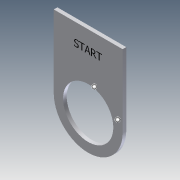
# Autodesk Inventor part: Start Button Lable
Saved by Autodesk Inventor 2016 (Build 200138000, 138)
## iProperties
Created: 2005-06-20
Part Number: Start Button Lable
Checked By: ~
Material: Generic
Document SubType Name: Modeling
Designer: BassBW
Manufacturer: Standard
Standards Organization: Custom
Density: 1 g/cm^3
Appearance: White
SCALE: 1:1
STOCK SIZE: SEE DWG
UNITS: ANSI
COMMODITY: MFG
Author: BassBW
Autodesk Inventor part; units mm, degrees
ref_plane "YZ Plane" through (0, 0, 0) normal (1, 0, 0) x (0, 1, 0)
ref_plane "XZ Plane" through (0, 0, 0) normal (0, 1, 0) x (-1, 0, 0)
ref_plane "XY Plane" through (0, 0, 0) normal (0, 0, 1) x (1, 0, 0)
sketch "Sketch1" plane through (0, 0, 0) normal (0, 0, 1) x (1, 0, 0)
  line L0 (30.1625, 0) -> (30.1625, 31.75)
  line L1 (30.1625, 31.75) -> (0, 31.75)
  line L2 (0, 31.75) -> (0, 0)
  arc A0 (0, 0) -> (30.1625, 0) centre (15.0813, 0) ccw
  dimension "d34" = 30.1625
  dimension "d35" = 31.75
  constraints: 6 end point, 2 point on circle, 2 tangent, 1 centre point, 1 horizontal, 1 parallel, 1 vertical
  measures "d34" distance of L0.end L1.end
  measures "d35" distance from line of A0.centre L1
extrude "Extrusion6" add sketch "Sketch1" along normal blind 1.5875
sketch "Sketch9" plane through (0, 0, 1.5875) normal (0, 0, 1) x (1, 0, 0)
  arc A0 (0, 0) -> (30.1625, 0) centre (15.0813, 0) ccw projected
  circle A1 centre (15.0813, 0) radius 11
  dimension "d38" = 22
  constraints: 1 centre point, 1 coincident
  measures "d38" diameter of A1
extrude "Extrusion7" cut sketch "Sketch9" against normal through all
sketch "Sketch10" plane through (0, 0, 1.5875) normal (0, 0, 1) x (1, 0, 0)
  line L0 (8.7312, 25.4) -> (21.4312, 25.4) construction
  line L1 (21.4312, 25.4) -> (21.4312, 22.225) construction
  line L2 (21.4312, 22.225) -> (8.7312, 22.225) construction
  line L3 (8.7312, 22.225) -> (8.7312, 25.4) construction
  circle A0 centre (15.0813, 0) radius 11 projected
  spline S0 degree 3 poles (9.8897, 22.2433) (9.5587, 22.2433) (9.0943, 22.3816) (8.8893, 22.4804) knots 0 0 0 0 1 1 1 1
  line L4 (8.8893, 22.4804) -> (8.8893, 22.9893)
  line L5 (8.8893, 22.9893) -> (8.919, 22.9893)
  spline S1 degree 3 poles (8.919, 22.9893) (9.119, 22.8015) (9.6254, 22.5941) (9.86, 22.5941) knots 0 0 0 0 1 1 1 1
  spline S2 degree 3 poles (9.86, 22.5941) (10.196, 22.5941) (10.5393, 22.8732) (10.5393, 23.1029) knots 0 0 0 0 1 1 1 1
  spline S3 degree 3 poles (10.5393, 23.1029) (10.5393, 23.2857) (10.359, 23.5129) (10.1639, 23.5697) knots 0 0 0 0 1 1 1 1
  spline S4 degree 3 poles (10.1639, 23.5697) (10.0231, 23.6092) (9.7884, 23.6636) (9.613, 23.708) knots 0 0 0 0 1 1 1 1
  spline S5 degree 3 poles (9.613, 23.708) (9.455, 23.75) (9.2055, 23.876) (9.1092, 23.9773) knots 0 0 0 0 1 1 1 1
  spline S6 degree 3 poles (9.1092, 23.9773) (9.0153, 24.0785) (8.9116, 24.3502) (8.9116, 24.5281) knots 0 0 0 0 1 1 1 1
  spline S7 degree 3 poles (8.9116, 24.5281) (8.9116, 24.8986) (9.4895, 25.4) (9.9366, 25.4) knots 0 0 0 0 1 1 1 1
  spline S8 degree 3 poles (9.9366, 25.4) (10.1935, 25.4) (10.648, 25.2987) (10.8431, 25.2024) knots 0 0 0 0 1 1 1 1
  line L6 (10.8431, 25.2024) -> (10.8431, 24.7183)
  line L7 (10.8431, 24.7183) -> (10.8135, 24.7183)
  spline S9 degree 3 poles (10.8135, 24.7183) (10.6677, 24.8517) (10.2133, 25.0493) (9.9638, 25.0493) knots 0 0 0 0 1 1 1 1
  spline S10 degree 3 poles (9.9638, 25.0493) (9.6822, 25.0493) (9.3339, 24.785) (9.3339, 24.5701) knots 0 0 0 0 1 1 1 1
  spline S11 degree 3 poles (9.3339, 24.5701) (9.3339, 24.3774) (9.5389, 24.1477) (9.7316, 24.0958) knots 0 0 0 0 1 1 1 1
  spline S12 degree 3 poles (9.7316, 24.0958) (9.86, 24.0613) (10.233, 23.9723) (10.3565, 23.9353) knots 0 0 0 0 1 1 1 1
  spline S13 degree 3 poles (10.3565, 23.9353) (10.6702, 23.8389) (10.9617, 23.4512) (10.9617, 23.1671) knots 0 0 0 0 1 1 1 1
  spline S14 degree 3 poles (10.9617, 23.1671) (10.9617, 22.9868) (10.8159, 22.641) (10.685, 22.52) knots 0 0 0 0 1 1 1 1
  spline S15 degree 3 poles (10.685, 22.52) (10.5393, 22.3866) (10.1688, 22.2433) (9.8897, 22.2433) knots 0 0 0 0 1 1 1 1
  line L8 (12.0855, 22.2977) -> (12.0855, 24.985)
  line L9 (12.0855, 24.985) -> (11.0629, 24.985)
  line L10 (11.0629, 24.985) -> (11.0629, 25.3457)
  line L11 (11.0629, 25.3457) -> (13.5132, 25.3457)
  line L12 (13.5132, 25.3457) -> (13.5132, 24.985)
  line L13 (13.5132, 24.985) -> (12.4906, 24.985)
  line L14 (12.4906, 24.985) -> (12.4906, 22.2977)
  line L15 (12.4906, 22.2977) -> (12.0855, 22.2977)
  line L16 (13.4934, 22.2977) -> (14.521, 25.3457)
  line L17 (14.521, 25.3457) -> (15.0199, 25.3457)
  line L18 (15.0199, 25.3457) -> (16.0474, 22.2977)
  line L19 (16.0474, 22.2977) -> (15.6201, 22.2977)
  line L20 (15.6201, 22.2977) -> (15.3435, 23.1498)
  line L21 (15.3435, 23.1498) -> (14.1801, 23.1498)
  line L22 (14.1801, 23.1498) -> (13.9035, 22.2977)
  line L23 (13.9035, 22.2977) -> (13.4934, 22.2977)
  line L24 (15.2323, 23.4956) -> (14.7606, 24.9307)
  line L25 (14.7606, 24.9307) -> (14.2913, 23.4956)
  line L26 (14.2913, 23.4956) -> (15.2323, 23.4956)
  line L27 (18.6953, 22.2977) -> (18.1692, 22.2977)
  line L28 (18.1692, 22.2977) -> (17.2059, 23.5104)
  line L29 (17.2059, 23.5104) -> (16.7415, 23.5104)
  line L30 (16.7415, 23.5104) -> (16.7415, 22.2977)
  line L31 (16.7415, 22.2977) -> (16.3364, 22.2977)
  line L32 (16.3364, 22.2977) -> (16.3364, 25.3457)
  line L33 (16.3364, 25.3457) -> (17.1219, 25.3457)
  spline S16 degree 3 poles (17.1219, 25.3457) (17.3837, 25.3457) (17.7369, 25.2888) (17.8975, 25.1851) knots 0 0 0 0 1 1 1 1
  spline S17 degree 3 poles (17.8975, 25.1851) (18.058, 25.0814) (18.2433, 24.7578) (18.2433, 24.5182) knots 0 0 0 0 1 1 1 1
  spline S18 degree 3 poles (18.2433, 24.5182) (18.2433, 24.1848) (17.9024, 23.7327) (17.611, 23.6241) knots 0 0 0 0 1 1 1 1
  line L34 (17.611, 23.6241) -> (18.6953, 22.2977)
  spline S19 degree 3 poles (17.8209, 24.4861) (17.8209, 24.6195) (17.727, 24.8245) (17.6282, 24.8912) knots 0 0 0 0 1 1 1 1
  spline S20 degree 3 poles (17.6282, 24.8912) (17.5418, 24.948) (17.3121, 24.9949) (17.1441, 24.9949) knots 0 0 0 0 1 1 1 1
  line L35 (17.1441, 24.9949) -> (16.7415, 24.9949)
  line L36 (16.7415, 24.9949) -> (16.7415, 23.8488)
  line L37 (16.7415, 23.8488) -> (17.0972, 23.8488)
  spline S21 degree 3 poles (17.0972, 23.8488) (17.2726, 23.8488) (17.5517, 23.9106) (17.648, 24.0069) knots 0 0 0 0 1 1 1 1
  spline S22 degree 3 poles (17.648, 24.0069) (17.7369, 24.0909) (17.8209, 24.328) (17.8209, 24.4861) knots 0 0 0 0 1 1 1 1
  line L38 (19.6487, 22.2977) -> (19.6487, 24.985)
  line L39 (19.6487, 24.985) -> (18.6261, 24.985)
  line L40 (18.6261, 24.985) -> (18.6261, 25.3457)
  line L41 (18.6261, 25.3457) -> (21.0764, 25.3457)
  line L42 (21.0764, 25.3457) -> (21.0764, 24.985)
  line L43 (21.0764, 24.985) -> (20.0538, 24.985)
  line L44 (20.0538, 24.985) -> (20.0538, 22.2977)
  line L45 (20.0538, 22.2977) -> (19.6487, 22.2977)
  dimension "d41" = 3.175
  dimension "d42" = 12.7
  dimension "d43" = 22.225
  dimension "d44" = 6.35
  constraints: 2 other
  measures "d41" distance between parallel lines of L0 L2
  measures "d42" distance between parallel lines of L1 L3
  measures "d43" distance from line of A0.centre L2
  measures "d44" distance from line of A0.centre L3
emboss "Emboss2" sketch "Sketch10" operation cut depth 0.1778 direction (0, 0, -1) contours S0 L4 L5 S1 S2 S3 S4 S5 S6 S7 S8 L6 L7 S9 S10 S11 S12 S13 S14 S15 | L8 L9 L10 L11 L12 L13 L14 L15 | L16 L17 L18 L19 L20 L21 L22 L23 | L27 L28 L29 L30 L31 L32 L33 S16 S17 S18 L34 | L38 L39 L40 L41 L42 L43 L44 L45
equation "\"d44\" = 0.5 * d42"
body "Solid1"
